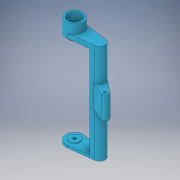
# Autodesk Inventor part: Servo-Arm-Lip
Saved by Autodesk Inventor 2018.3 (Build 223284000, 284)
## iProperties
Created: 2018-02-17
Part Number: Servo-Arm-Lip
Material: Generisch
Document SubType Name: Modeling
Designer: JochenAlt
Density: 1 g/cm^3
Appearance: Vorgabe
Author: JochenAlt
Autodesk Inventor part; units mm, degrees
ref_plane "YZ Plane" through (0, 0, 0) normal (1, 0, 0) x (0, 1, 0)
ref_plane "XZ Plane" through (0, 0, 0) normal (0, 1, 0) x (-1, 0, 0)
sketch "Skizze1" plane through (0, 0, 0) normal (0, 0, 1) x (1, 0, 0)
  line L0 (0, 5.6) -> (0, -5.6) construction
  line L1 (-9.12, 0) -> (26.72, 0) construction
  circle A0 centre (0, 0) radius 2
  circle A1 centre (9.5, 0) radius 1
  circle A2 centre (16, 0) radius 1
  circle A3 centre (19, 0) radius 1
  arc A4 (19.1916, -2.5929) -> (19.1916, 2.5929) centre (19, 0) ccw
  arc A5 (0.2947, 3.9891) -> (0.2947, -3.9891) centre (0, 0) ccw
  line L2 (0.2947, 3.9891) -> (19.1916, 2.5929)
  line L3 (0.2947, -3.9891) -> (19.1916, -2.5929)
  circle A6 centre (12.8, 0) radius 1
  circle A7 centre (0, 0) radius 4
  point P0 (0.5263, 3.9652)
  point P1 (0.6579, -1.8887)
  point P2 (0.6579, 1.8887)
  dimension "d0" = 9.5
  dimension "d1" = 16
  dimension "d2" = 19
  dimension "d3" = 5.2
  dimension "d4" = 2
  dimension "d5" = 4
  dimension "d6" = 8
  dimension "d17" = 12.8
  constraints: 7 centre point, 7 point on circle, 4 coincident, 4 end point, 4 point on line, 4 tangent, 3 equal radius, 3 other
  measures "d0" distance of A1.centre point (0, 0)
  measures "d1" distance of point (0, 0) A2.centre
  measures "d2" distance of A3.centre point (0, 0)
  measures "d3" diameter of A4
  measures "d4" diameter of A3
  measures "d5" diameter of A0
  measures "d6" diameter of A5
  measures "d17" distance of A6.centre point (0, 0)
extrude "Extrusion1" add sketch "Skizze1" along normal blind 1.8
extrude "Extrusion2" add sketch "Skizze1" against normal blind 2.7 contours A5 A7
sketch "Skizze6" plane through (0, 0, 0) normal (0, 0, 1) x (1, 0, 0)
  line L0 (0.2947, 3.9891) -> (19.1916, 2.5929) construction
  arc A0 (19.1916, -2.5929) -> (19.1916, 2.5929) centre (19, 0) ccw construction
  line L1 (19.1916, -2.5929) -> (0.2947, -3.9891) construction
  arc A1 (0.2947, -3.9891) -> (0.2947, 3.9891) centre (0, 0) ccw construction
  circle A2 centre (12.8, 0) radius 1 construction
  circle A3 centre (19, 0) radius 1 construction
  circle A4 centre (16, 0) radius 1 construction
  circle A5 centre (9.5, 0) radius 1 construction
  arc A6 (19.1989, -2.6927) -> (19.1989, 2.6927) centre (19, 0) ccw
  line L2 (19.1989, 2.6927) -> (0.3021, 4.0889)
  circle A7 centre (9.5, 0) radius 1 construction
  circle A8 centre (19, 0) radius 1
  line L3 (-14.3, 0) -> (40.3, 0) construction
  line L4 (0.3021, -4.0889) -> (19.1989, -2.6927)
  circle A9 centre (0, 0) radius 2 construction
  circle A10 centre (0, 0) radius 1.25
  arc A11 (0.7868, 6.4522) -> (0.7868, -6.4522) centre (0, 0) ccw
  line L5 (19, 0) -> (29.3937, -6.0008) construction
  circle A12 centre (29.3937, -6.0008) radius 1.15
  circle A13 centre (29.3937, -6.0008) radius 2.5
  arc A14 (15.9906, -2.9297) -> (15.9906, 2.9297) centre (19, 0) ccw
  line L6 (17.4364, -3.8981) -> (28.463, -8.3211)
  line L7 (21.594, 3.3032) -> (30.9378, -4.0346)
  line L8 (0.7868, -6.4522) -> (19.5084, -4.1691)
  arc A15 (15.9906, 2.9297) -> (15.9906, -2.9297) centre (19, 0) ccw
  line L9 (15.9906, -2.9297) -> (16.191, -4.5737)
  line L10 (19.5084, 4.1691) -> (0.7868, 6.4522)
  line L11 (16.191, 4.5737) -> (15.9906, 2.9297)
  line L12 (29.3937, -6.0008) -> (0, 0) construction
  arc A16 (0.3021, 4.0889) -> (0.3021, -4.0889) centre (0, 0) ccw
  arc A17 (0.3021, -4.0889) -> (0.3021, 4.0889) centre (0, 0) ccw
  dimension "d106" = 2.5
  dimension "d116" = 0.1
  dimension "d235" = 6.5
  dimension "d250" = 2.3
  dimension "d251" = 5
  dimension "d252" = 150
  dimension "d253" = 1.5
  dimension "d261" = 30
  constraints: 20 end point, 18 point on circle, 12 centre point, 11 tangent, 8 coincident, 4 point on line, 2 concentric, 2 perpendicular, 1 parallel
  measures "d106" diameter of A10
  measures "d116" distance between parallel lines of L4 L1
  measures "d235" radius of A11
  measures "d250" diameter of A12
  measures "d251" diameter of A13
  measures "d252" angle of L3 L5
  measures "d253" radial gap between concentric circles of A14 A6
  measures "d261" distance of L12.end L12.start
extrude "Extrusion11" add sketch "Skizze6" along normal blind 2 separate body contours A6 L2 A14 L4 | L9 L8 A11 L10 L11 L2 A16 L4 | A14 L6 L8 L9 | L11 L10 A14 | A14 L8 L6
extrude "Extrusion12" add sketch "Skizze6" along normal blind 1.5 from surface at 2 contours L4 A15 L2 A6 | A6 L2 A14 L4 | L9 L8 A11 L10 L11 L2 A16 L4 | L4 A17 L2 A15 | A14 L6 L8 L9 | L11 L10 A14 | A16 A17 | A14 L8 L6 | A8 bodies 2
sketch "Skizze18" plane through (0, 0, 3.5) normal (0, 0, 1) x (0.9999808, 0.0061906, 0)
  circle A0 centre (0, 0) radius 5.15
  circle A1 centre (0, 0) radius 6.5
  circle A2 centre (0, 0) radius 4
  line L0 (19.4822, -4.2898) -> (0.7469, -6.4569) construction
  arc A3 (19.4822, -4.2898) -> (19.5339, 4.0483) centre (18.9996, -0.1176) ccw construction
  line L1 (0.8268, 6.4472) -> (19.5339, 4.0483) construction
  arc A4 (0.8268, 6.4472) -> (0.7469, -6.4569) centre (0, 0) ccw construction
  point P0 (-6.4999, 0.0402)
  dimension "d183" = 10.3
  dimension "d192" = 8
  constraints: 3 coincident, 2 centre point, 1 point on circle, 3 other
  measures "d183" diameter of A0
  measures "d192" diameter of A2
extrude "Extrusion29" add sketch "Skizze18" along normal blind 3 contours A0 | A1 bodies 2
extrude "Extrusion28" add sketch "Skizze18" along normal blind 4 from surface at 3 contours A1 bodies 2
extrude "Extrusion37" add sketch "Skizze6" against normal blind 70 contours A6 L2 A14 L4 | A14 L6 L8 L9 | L11 L10 A14 | A14 L8 L6 bodies 2
extrude "Extrusion34" add sketch "Skizze6" against normal blind 2 from surface at -70 contours L4 A15 L2 A6 | A6 L2 A14 L4 | L9 L8 A11 L10 L11 L2 A16 L4 | L4 A17 L2 A15 | A14 L6 L8 L9 | L11 L10 A14 | A16 A17 | A14 L8 L6 | A8 bodies 2
extrude "Extrusion35" add sketch "Skizze6" along normal blind 0.5 from surface at -70 contours A16 A17 bodies 2
ref_plane "Arbeitsebene10" through (0, 0, -30) normal (0, 0, 1) x (1, 0, 0)
extrude "Extrusion36" add sketch "Skizze6" along normal mid plane 17 from surface at -30 contours A14 L8 L6 | A14 L7 A13 L6 L8 | A13 bodies 2
sketch "Skizze23" plane through (17.4364, -3.8981, -30) normal (0, 0, 1) x (0.9281172, -0.3722882, 0)
  line L0 (-1.7024, 0.3605) -> (-0.9043, -1.0906) projected
  line L1 (-14.5019, -8.5689) -> (-0.9043, -1.0906) projected
  arc A0 (-19.306, 3.4079) -> (-14.5019, -8.5689) centre (-17.6342, -2.8735) ccw projected
  line L2 (-4.3098, 7.3992) -> (-19.306, 3.4079) projected
  line L3 (-4.3098, 7.3992) -> (-3.8838, 5.7987) projected
  line L4 (-18.8761, 1.0339) -> (-3.8838, 5.7987) projected
  line L5 (-1.7024, 0.3605) -> (-15.8316, -6.5559) projected
  line L6 (-0.8178, 6.7732) -> (-3.8838, 5.7987) projected
  line L7 (0.3275, 8.6334) -> (-4.3098, 7.3992)
  arc A1 (1.1871, 1.775) -> (-0.8178, 6.7732) centre (0, 4.2) ccw projected
  line L8 (0.1989, 6.8927) -> (0.3275, 8.6334)
  arc A2 (-18.8761, 1.0339) -> (-15.8316, -6.5559) centre (-17.6342, -2.8735) ccw projected
  constraints: 4 end point, 1 collinear, 1 point on circle
extrude "Extrusion40" cut sketch "Skizze23" along normal mid plane 7 bodies 2
